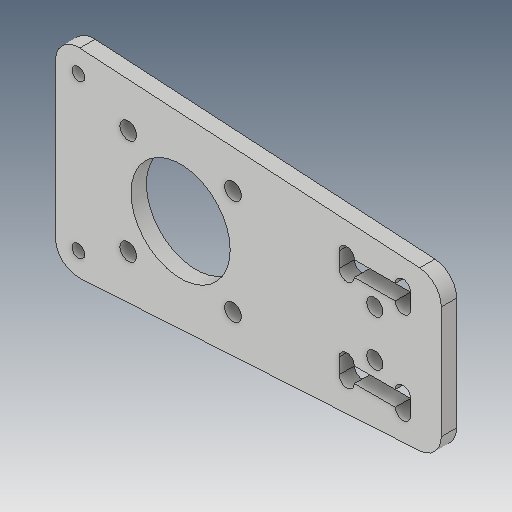
# Autodesk Inventor part: BaseSliderMount
Saved by Autodesk Inventor 2019.4 (Build 234330000, 330)
## iProperties
Created: 2019-07-01
Part Number: BaseSliderMount
Material: Generic
Document SubType Name: Modeling
Designer: AzLIer
Density: 1 g/cm^3
Appearance: Default
Author: AzLIer
Autodesk Inventor part; units mm, degrees
ref_plane "YZ Plane" through (0, 0, 0) normal (1, 0, 0) x (0, 1, 0)
ref_plane "XZ Plane" through (0, 0, 0) normal (0, 1, 0) x (-1, 0, 0)
ref_plane "XY Plane" through (0, 0, 0) normal (0, 0, 1) x (1, 0, 0)
sketch "スケッチ1" plane through (0, 0, 0) normal (0, 0, 1) x (1, 0, 0)
  circle A0 centre (0, 15) radius 1.25
  circle A1 centre (0, -15) radius 1.25
  circle A2 centre (20, 0) radius 9.7
  line L0 (0, 15) -> (0, -15) construction
  line L1 (72.6, 25) -> (-7.4, 25)
  line L2 (-7.4, 25) -> (-7.4, -25)
  line L3 (-7.4, -25) -> (72.6, -25)
  line L4 (72.6, -25) -> (72.6, 25)
  circle A3 centre (9.747, 10.253) radius 1.65
  circle A4 centre (9.747, -10.253) radius 1.65
  circle A5 centre (30.253, -10.253) radius 1.65
  circle A6 centre (30.253, 10.253) radius 1.65
  line L5 (62, 7.5) -> (54, 7.5)
  line L6 (51, 7.5) -> (51, 10.5)
  line L7 (54, 10.5) -> (62, 10.5)
  line L8 (65, 10.5) -> (65, 7.5)
  arc A7 (62, 7.5) -> (65, 7.5) centre (63.5, 7.5) ccw
  arc A8 (65, 10.5) -> (62, 10.5) centre (63.5, 10.5) ccw
  arc A9 (51, 7.5) -> (54, 7.5) centre (52.5, 7.5) ccw
  arc A10 (54, 10.5) -> (51, 10.5) centre (52.5, 10.5) ccw
  line L9 (20, 0) -> (0, 0) construction
  line L10 (62, -7.5) -> (54, -7.5)
  line L11 (51, -7.5) -> (51, -10.5)
  line L12 (54, -10.5) -> (62, -10.5)
  line L13 (65, -10.5) -> (65, -7.5)
  arc A11 (65, -7.5) -> (62, -7.5) centre (63.5, -7.5) ccw
  arc A12 (62, -10.5) -> (65, -10.5) centre (63.5, -10.5) ccw
  arc A13 (54, -7.5) -> (51, -7.5) centre (52.5, -7.5) ccw
  arc A14 (51, -10.5) -> (54, -10.5) centre (52.5, -10.5) ccw
  circle A15 centre (58, -4.5) radius 1.6
  circle A16 centre (58, 4.5) radius 1.6
  point P0 (-7.4, 0)
  point P1 (58, 7.5)
  dimension "d0" = 2.5
  dimension "d1" = 30
  dimension "d2" = 19.4
  dimension "d4" = 7.4
  dimension "d5" = 50
  dimension "d6" = 80
  dimension "d9" = 3.3
  dimension "d11" = 14.5
  dimension "d14" = 360
  dimension "d18" = 14
  dimension "d19" = 3
  dimension "d20" = 10.5
  dimension "d21" = 51
  dimension "d22" = 1.5
  dimension "d23" = 3.2
  dimension "d24" = 3.2
  dimension "d25" = 3
  dimension "d26" = 3
  dimension "d36" = 20
  constraints: 28 end point, 17 centre point, 16 point on circle, 16 point on line, 12 symmetric about line, 4 equal radius, 4 parallel, 3 horizontal, 3 midpoint, 3 vertical alignment, 2 coincident, 2 horizontal alignment, 2 perpendicular, 1 vertical, 13 other
  measures "d0" diameter of A0
  measures "d1" distance of L0.start L0.end
  measures "d2" diameter of A2
  measures "d4" distance from line of point (0, 0) L2
  measures "d5" distance of L3.end L1.start
  measures "d6" distance from line of point (-7.4, 0) L4
  measures "d9" diameter of A3
  measures "d11" distance of L9.start A3.centre
  measures "d18" distance of L6.end L8.start
  measures "d19" distance of L8.start L8.end
  measures "d20" distance from line of L9.start L7
  measures "d21" distance from line of L6 point (0, 0)
  measures "d22" radius of A10
  measures "d23" diameter of A15
  measures "d24" diameter of A16
  measures "d25" distance from line of L10 A15.centre
  measures "d26" distance from line of L5 A16.centre
  measures "d36" distance of L9.end L9.start
extrude "押し出し1" add sketch "スケッチ1" along normal blind 3
sketch "スケッチ3" plane through (0, 0, 0) normal (0, 0, -1) x (-1, 0, 0)
  circle A0 centre (-20, 0) radius 9.7 projected
  arc A1 (-65, 7.5) -> (-62, 7.5) centre (-63.5, 7.5) ccw projected
  line L0 (-65, 7.5) -> (-65, 10.5) projected
  line L1 (-62, 10.5) -> (-54, 10.5) projected
  arc A2 (-51, 10.5) -> (-54, 10.5) centre (-52.5, 10.5) ccw projected
  line L2 (-51, 10.5) -> (-51, 7.5) projected
  arc A3 (-54, 7.5) -> (-51, 7.5) centre (-52.5, 7.5) ccw projected
  line L3 (-54, 7.5) -> (-62, 7.5) projected
  arc A4 (-51, -7.5) -> (-54, -7.5) centre (-52.5, -7.5) ccw projected
  line L4 (-51, -7.5) -> (-51, -10.5) projected
  arc A5 (-54, -10.5) -> (-51, -10.5) centre (-52.5, -10.5) ccw projected
  line L5 (-54, -10.5) -> (-62, -10.5) projected
  line L6 (-65, -10.5) -> (-65, -7.5) projected
  arc A6 (-62, -7.5) -> (-65, -7.5) centre (-63.5, -7.5) ccw projected
  line L7 (-62, -7.5) -> (-54, -7.5) projected
  circle A7 centre (-30.253, 10.253) radius 1.65 projected
  circle A8 centre (-30.253, -10.253) radius 1.65 projected
  circle A9 centre (-9.747, -10.253) radius 1.65 projected
  circle A10 centre (-9.747, 10.253) radius 1.65 projected
  circle A11 centre (-58, 4.5) radius 1.6 projected
  circle A12 centre (-58, -4.5) radius 1.6 projected
  circle A13 centre (0, -15) radius 1.25 projected
  circle A14 centre (0, 15) radius 1.25 projected
  line L8 (-72.6, 25) -> (7.4, 25) projected
  line L9 (-72.6, -25) -> (-72.6, 25) projected
  line L10 (7.4, -25) -> (-72.6, -25) projected
  line L11 (7.4, 25) -> (7.4, -25) projected
  arc A15 (-71, -11) -> (-66.7702, -15.4919) centre (-66.5, -11) ccw
  arc A16 (-66.7702, 15.4919) -> (-71, 11) centre (-66.5, 11) ccw
  line L12 (-71, -11) -> (-71, 11)
  arc A17 (-0.2702, -19.4919) -> (4.5, -15) centre (0, -15) ccw
  arc A18 (4.5, 15) -> (-0.2702, 19.4919) centre (0, 15) ccw
  line L13 (-66.7702, -15.4919) -> (-0.2702, -19.4919)
  line L14 (4.5, -15) -> (4.5, 15)
  line L15 (-0.2702, 19.4919) -> (-66.7702, 15.4919)
  line L16 (0, 0) -> (-20, 0) construction
  arc A19 (-62, 10.5) -> (-65, 10.5) centre (-63.5, 10.5) ccw projected
  arc A20 (-65, -10.5) -> (-62, -10.5) centre (-63.5, -10.5) ccw projected
  dimension "d29" = 9
  dimension "d30" = 9
  dimension "d31" = 4.5
  dimension "d32" = 22
  dimension "d33" = 6
  constraints: 10 end point, 8 point on circle, 8 tangent, 4 centre point, 2 coincident, 1 equal radius, 1 horizontal, 1 symmetric about line, 1 vertical alignment
  measures "d29" diameter of A17
  measures "d30" diameter of A18
  measures "d31" radius of A16
  measures "d32" distance of A16.centre A15.centre
  measures "d33" distance between parallel lines of L6 L12
extrude "押し出し2" cut sketch "スケッチ3" against normal blind 3 contours L8 L11 L10 L9
